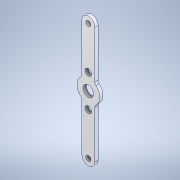
# Autodesk Inventor part: EncoderStrip
Saved by Autodesk Inventor 2020 (Build 240168000, 168)
## iProperties
Created: 2019-06-24
Part Number: EncoderStrip
Material: Aluminum 6061
Document SubType Name: Modeling
Designer: Connor
Density: 2.7 g/cm^3
Appearance: Aluminum - Flat
Author: Connor
Autodesk Inventor part; units mm, degrees
ref_plane "YZ Plane" through (0, 0, 0) normal (1, 0, 0) x (0, 1, 0)
ref_plane "XZ Plane" through (0, 0, 0) normal (0, 1, 0) x (-1, 0, 0)
ref_plane "XY Plane" through (0, 0, 0) normal (0, 0, 1) x (1, 0, 0)
sketch "Sketch1" plane through (0, 0, 0) normal (0, 0, 1) x (1, 0, 0)
  line L0 (0, -57.15) -> (0, 57.15) construction
  line L1 (6.35, -57.15) -> (6.35, 57.15)
  line L2 (-6.35, 57.15) -> (-6.35, -57.15)
  arc A0 (-6.35, -57.15) -> (6.35, -57.15) centre (0, -57.15) ccw
  arc A1 (6.35, 57.15) -> (-6.35, 57.15) centre (0, 57.15) ccw
  circle A2 centre (0, 57.15) radius 2.4892
  circle A3 centre (0, -57.15) radius 2.4892
  circle A4 centre (0, 0) radius 5.1562
  circle A5 centre (0, 0) radius 11.1125
  point P0 (-6.35, 9.1195)
  point P1 (-6.35, -9.1195)
  point P2 (6.35, -9.1195)
  point P3 (6.35, 9.1195)
  dimension "d0" = 114.3
  dimension "d1" = 12.7
  dimension "d2" = 4.9784
  dimension "d3" = 10.3124
  dimension "d4" = 22.225
  constraints: 8 end point, 6 centre point, 4 coincident, 4 point on circle, 4 tangent, 1 equal radius, 1 midpoint, 1 parallel, 1 vertical
  measures "d0" distance of L0.start L0.end
  measures "d1" distance between parallel lines of L1 L2
  measures "d2" diameter of A2
  measures "d3" diameter of A4
  measures "d4" diameter of A5
extrude "Extrusion1" add sketch "Sketch1" along normal blind 3.175
sketch "Sketch2" plane through (0, 0, 3.175) normal (0, 0, 1) x (1, 0, 0)
  circle A0 centre (0, 0) radius 15.875 construction
  circle A1 centre (0, 15.875) radius 3.175
  circle A2 centre (0, -15.875) radius 3.175
  dimension "d7" = 31.75
  dimension "d8" = 6.35
  dimension "d9" = 6.35
  constraints: 3 centre point, 2 point on circle, 2 vertical alignment, 1 coincident
  measures "d7" diameter of A0
  measures "d8" diameter of A1
  measures "d9" diameter of A2
extrude "Extrusion2" cut sketch "Sketch2" against normal through all
fillet "Fillet1" radius 3.175 4 edges at (6.35, 9.1195, 1.5875) (6.35, -9.1195, 1.5875) (-6.35, -9.1195, 1.5875) (-6.35, 9.1195, 1.5875)
body "Solid1"
